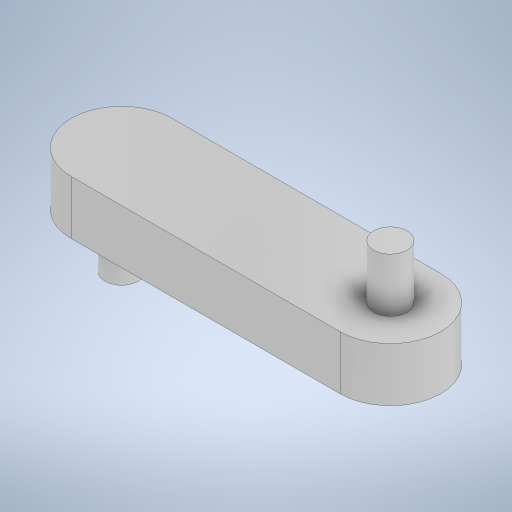
# Autodesk Inventor part: Connecting_bar
Saved by Autodesk Inventor 2024 (Build 280153000, 153)
## iProperties
Created: 2023-10-06
Part Number: Connecting_bar
Material: Generic
Document SubType Name: Modeling
Designer: tangl
Density: 1 g/cm^3
Appearance: Aluminum - Polished
Author: tangl
Autodesk Inventor part; units mm, degrees
ref_plane "YZ Plane" through (0, 0, 0) normal (1, 0, 0) x (0, 1, 0)
ref_plane "XZ Plane" through (0, 0, 0) normal (0, 1, 0) x (-1, 0, 0)
ref_plane "XY Plane" through (0, 0, 0) normal (0, 0, 1) x (1, 0, 0)
sketch "Sketch1" plane through (0, 0, 0) normal (0, 1, 0) x (-1, 0, 0)
  line L0 (0, 0) -> (50.8, 0) construction
  arc A0 (0, 9.525) -> (0, -9.525) centre (0, 0) ccw
  line L1 (0, -9.525) -> (50.8, -9.525)
  line L2 (0, 9.525) -> (50.8, 9.525)
  circle A1 centre (50.8, 0) radius 9.525
  dimension "d1" = 50.8
  dimension "d4" = 19.05
  dimension "d14" = 50.8
  dimension "d15" = 50.8
  dimension "d16" = 19.05
  constraints: 6 end point, 3 coincident, 3 horizontal, 3 point on circle, 1 centre point, 3 other
  measures "d1" distance of L0.start L0.end
  measures "d4" diameter of A0
  measures "d14" distance of L1.start L1.end
  measures "d15" distance of L2.start L2.end
  measures "d16" distance between parallel lines of L2 L1
extrude "Extrusion1" add sketch "Sketch1" along normal blind 10.16
sketch "Sketch4" plane through (0, 10.16, 0) normal (0, 1, 0) x (1, 0, 0)
  circle A0 centre (0, 0) radius 3.175
  dimension "d17" = 6.35
  constraints: 1 centre point, 1 coincident
  measures "d17" diameter of A0
extrude "Extrusion4" add sketch "Sketch4" along normal blind 10.16
sketch "Sketch5" plane through (0, 0, 0) normal (0, -1, 0) x (1, 0, 0)
  circle A0 centre (-50.8, 0) radius 3.175
  arc A1 (-50.8, 9.525) -> (-50.8, -9.525) centre (-50.8, 0) ccw projected
  point P0 (0, 0)
  dimension "d20" = 6.35
  constraints: 1 centre point, 1 concentric
  measures "d20" diameter of A0
extrude "Extrusion5" add sketch "Sketch5" along normal blind 10.16
body "Solid1"
